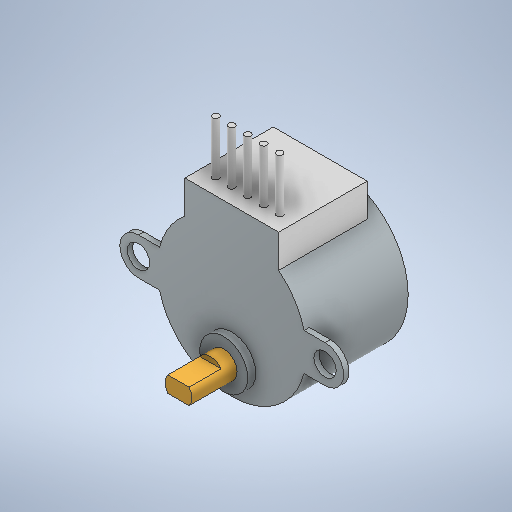
# Autodesk Inventor part: 28BYJ-48
Saved by Autodesk Inventor 2025 (Build 290162000, 162)
## iProperties
Created: 2025-07-13
Part Number: 28BYJ-48
Material: 一般
Document SubType Name: Modeling
Designer: daisuke
Density: 1 g/cm^3
Appearance: 既定
Author: daisuke
Autodesk Inventor part; units mm, degrees
ref_plane "YZ Plane" through (0, 0, 0) normal (1, 0, 0) x (0, 1, 0)
ref_plane "XZ Plane" through (0, 0, 0) normal (0, 1, 0) x (-1, 0, 0)
ref_plane "XY Plane" through (0, 0, 0) normal (0, 0, 1) x (1, 0, 0)
sketch "スケッチ2" plane through (0, 0, 0) normal (0, 0, 1) x (1, 0, 0)
  circle A0 centre (0, 0) radius 14
  dimension "d0" = 28
  constraints: 1 centre point, 1 coincident
  measures "d0" diameter of A0
extrude "本体" add sketch "スケッチ2" along normal blind 19.1
sketch "スケッチ3" plane through (0, 0, 19.1) normal (0, 0, 1) x (1, 0, 0)
  line L0 (0, 16.0197) -> (0, -16.0197) construction
  line L1 (-23.6697, 0) -> (23.6697, 0) construction
  circle A0 centre (-17.5, 0) radius 2.1
  circle A1 centre (17.5, 0) radius 2.1
  circle A2 centre (-17.5, 0) radius 3.5
  circle A3 centre (17.5, 0) radius 3.5
  line L2 (-17.5, 3.5) -> (17.5, 3.5)
  line L3 (17.5, -3.5) -> (-17.5, -3.5)
  point P0 (0, 0)
  point P1 (0, 0)
  dimension "d3" = 4.2
  dimension "d4" = 35
  dimension "d5" = 7
  constraints: 8 end point, 4 centre point, 4 point on circle, 3 coincident, 2 equal radius, 2 midpoint, 2 point on line, 2 tangent, 1 horizontal, 1 parallel, 1 perpendicular, 1 symmetric about line, 1 vertical
  measures "d3" diameter of A0
  measures "d4" distance of A1.centre A0.centre
  measures "d5" diameter of A2
extrude "タブ" add sketch "スケッチ3" against normal blind 1
sketch "スケッチ4" plane through (0, 0, 19.1) normal (0, 0, 1) x (1, 0, 0)
  circle A0 centre (0, -8) radius 4.5
  point P0 (0, 0)
  dimension "d8" = 9
  dimension "d9" = 8
  constraints: 1 centre point, 1 vertical alignment
  measures "d8" diameter of A0
  measures "d9" distance of A0.centre point (0, 0)
extrude "押し出し3" add sketch "スケッチ4" along normal blind 1.5
sketch "スケッチ5" plane through (0, -8, 20.6) normal (0, 0, 1) x (1, 0, 0)
  circle A0 centre (0, 0) radius 2.5
  circle A1 centre (0, 0) radius 4.5 projected
  point P0 (0, 8)
  dimension "d12" = 5
  constraints: 1 centre point, 1 concentric
  measures "d12" diameter of A0
extrude "押し出し4" add sketch "スケッチ5" along normal blind 2.5 contours A0
sketch "スケッチ6" plane through (0, -8, 23.1) normal (0, 0, 1) x (1, 0, 0)
  circle A0 centre (0, 0) radius 2.5
  circle A1 centre (0, 0) radius 2.5 projected
  line L0 (-2.5, 1.5) -> (2.5, 1.5)
  line L1 (2.5, 1.5) -> (2.5, -1.5)
  line L2 (2.5, -1.5) -> (-2.5, -1.5)
  line L3 (-2.5, -1.5) -> (-2.5, 1.5)
  point P0 (0, 8)
  point P1 (2.5, 0)
  point P2 (0, 1.5)
  point P3 (-2, -1.5)
  point P4 (2, -1.5)
  point P5 (2, 1.5)
  point P6 (-2, 1.5)
  dimension "d15" = 3
  constraints: 8 end point, 2 concentric, 2 midpoint, 2 parallel, 1 centre point, 1 horizontal, 1 horizontal alignment, 1 perpendicular, 1 tangent, 1 vertical alignment
  measures "d15" distance of L0.end L1.end
extrude "押し出し5" add sketch "スケッチ6" along normal blind 6 contours A0 L2 L0
sketch "スケッチ7" plane through (0, 0, 19.1) normal (0, 0, 1) x (1, 0, 0)
  line L0 (-8.8, 0) -> (8.8, 0)
  line L1 (8.8, 0) -> (8.8, 17.1)
  line L2 (8.8, 17.1) -> (-8.8, 17.1)
  line L3 (-8.8, 17.1) -> (-8.8, 0)
  point P0 (0, 0)
  point P1 (0, 0)
  dimension "d18" = 17.6
  dimension "d19" = 17.1
  constraints: 8 end point, 2 parallel, 1 coincident, 1 horizontal, 1 midpoint, 1 perpendicular
  measures "d18" distance of L2.end L1.end
  measures "d19" distance of L0.end L1.end
extrude "押し出し6" add sketch "スケッチ7" against normal blind 16.6
sketch "スケッチ8" plane through (-8.8, 17.1, 19.1) normal (0, 1, 0) x (1, 0, 0)
  circle A0 centre (8.8, 3) radius 0.6
  line L0 (17.6, 0) -> (0, 0) projected
  point P0 (8.8, 19.1)
  dimension "d22" = 1.2
  dimension "d23" = 3
  constraints: 1 centre point, 1 vertical alignment
  measures "d22" diameter of A0
  measures "d23" distance from line of L0 A0.centre
extrude "押し出し7" add sketch "スケッチ8" along normal blind 10
pattern_linear "矩形状パターン1" count 5 spacing 3 along (-1, 0, 0) of "押し出し7" first direction both ways yes
